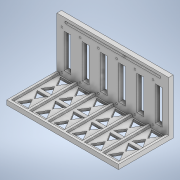
# Autodesk Inventor part: controllbox_1
Saved by Autodesk Inventor 2020 (Build 240168000, 168)
## iProperties
Created: 2020-05-26
Part Number: controllbox_1
Material: Generic
Document SubType Name: Modeling
Designer: Gebruiker
Density: 1 g/cm^3
Appearance: Default
Author: Gebruiker
Autodesk Inventor part; units mm, degrees
ref_plane "YZ Plane" through (0, 0, 0) normal (1, 0, 0) x (0, 1, 0)
ref_plane "XZ Plane" through (0, 0, 0) normal (0, 1, 0) x (-1, 0, 0)
ref_plane "XY Plane" through (0, 0, 0) normal (0, 0, 1) x (1, 0, 0)
sketch "Sketch1" plane through (0, 0, 0) normal (0, 0, 1) x (1, 0, 0)
  line L0 (-122.5, 60) -> (122.5, 60)
  line L1 (122.5, 60) -> (122.5, -60)
  line L2 (122.5, -60) -> (-122.5, -60)
  line L3 (-122.5, -60) -> (-122.5, 60)
  line L4 (-122.5, 60) -> (122.5, -60) construction
  line L5 (122.5, 60) -> (-122.5, -60) construction
  line L6 (-111.5, -60) -> (-111.5, 60) construction
  line L7 (-122.5, -47) -> (122.5, -47) construction
  circle A0 centre (-111.5, -47) radius 2
  circle A1 centre (-111.5, 39) radius 2
  line L8 (-111.5, 39) -> (122.5, 39) construction
  circle A2 centre (-71.5, -47) radius 2
  circle A3 centre (-31.5, -47) radius 2
  circle A4 centre (8.5, -47) radius 2
  circle A5 centre (48.5, -47) radius 2
  circle A6 centre (88.5, -47) radius 2
  line L9 (0, 60) -> (0, -60) construction
  circle A7 centre (-71.5, 39) radius 2
  circle A8 centre (-31.5, 39) radius 2
  circle A9 centre (8.5, 39) radius 2
  circle A10 centre (48.5, 39) radius 2
  circle A11 centre (88.5, 39) radius 2
  line L10 (-31.5, 39) -> (-31.5, -47) construction
  line L11 (-99.5, 60) -> (-99.5, -60) construction
  line L12 (-122.5, -4) -> (122.5, -4) construction
  line L13 (-107, 33.5) -> (-92, 33.5)
  line L14 (-92, 33.5) -> (-92, -41.5)
  line L15 (-92, -41.5) -> (-107, -41.5)
  line L16 (-107, -41.5) -> (-107, 33.5)
  line L17 (-107, 33.5) -> (-92, -41.5) construction
  line L18 (-92, 33.5) -> (-107, -41.5) construction
  line L19 (-67, 33.5) -> (-52, 33.5)
  line L20 (-52, 33.5) -> (-52, -41.5)
  line L21 (-67, -41.5) -> (-67, 33.5)
  line L22 (-52, -41.5) -> (-67, -41.5)
  line L23 (-27, 33.5) -> (-12, 33.5)
  line L24 (-12, 33.5) -> (-12, -41.5)
  line L25 (-27, -41.5) -> (-27, 33.5)
  line L26 (-12, -41.5) -> (-27, -41.5)
  line L27 (13, 33.5) -> (28, 33.5)
  line L28 (28, 33.5) -> (28, -41.5)
  line L29 (13, -41.5) -> (13, 33.5)
  line L30 (28, -41.5) -> (13, -41.5)
  line L31 (53, 33.5) -> (68, 33.5)
  line L32 (68, 33.5) -> (68, -41.5)
  line L33 (53, -41.5) -> (53, 33.5)
  line L34 (68, -41.5) -> (53, -41.5)
  line L35 (93, 33.5) -> (108, 33.5)
  line L36 (108, 33.5) -> (108, -41.5)
  line L37 (93, -41.5) -> (93, 33.5)
  line L38 (108, -41.5) -> (93, -41.5)
  line L39 (-105, 53.9067) -> (105, 53.9067)
  line L40 (105, 53.9067) -> (105, 48.9067)
  line L41 (105, 48.9067) -> (-105, 48.9067)
  line L42 (-105, 48.9067) -> (-105, 53.9067)
  line L43 (-105, 53.9067) -> (105, 48.9067) construction
  line L44 (105, 53.9067) -> (-105, 48.9067) construction
  point P0 (0, 0)
  point P1 (-99.5, -4)
  point P2 (0, 51.4067)
  dimension "d0" = 245
  dimension "d1" = 120
  dimension "d20" = 11
  dimension "d21" = 13
  dimension "d22" = 4
  dimension "d23" = 4
  dimension "d24" = 86
  dimension "d27" = 40
  dimension "d32" = 34
  dimension "d35" = 40
  dimension "d43" = 12
  dimension "d44" = 43
  dimension "d45" = 15
  dimension "d46" = 75
  dimension "d49" = 40
  dimension "d56" = 210
  dimension "d57" = 5
  constraints: 90 end point, 15 point on line, 12 centre point, 8 midpoint, 8 perpendicular, 6 horizontal, 6 parallel, 60 other
  measures "d0" distance of L1.end L2.end
  measures "d1" distance of L0.end L1.end
  measures "d20" distance between parallel lines of L6 L3
  measures "d21" distance between parallel lines of L7 L2
  measures "d22" diameter of A0
  measures "d23" diameter of A1
  measures "d24" distance of A0.centre L8.start
  measures "d27" distance of A0.centre A2.centre
  measures "d32" distance from line of L1 A6.centre
  measures "d35" distance of L8.start A7.centre
  measures "d43" distance from line of L11 L8.start
  measures "d44" distance from line of L12 L8.start
  measures "d45" distance of L14.end L15.end
  measures "d46" distance of L13.end L14.end
  measures "d49" distance of L13.start L19.start
  measures "d56" distance of L40.end L41.end
  measures "d57" distance of L39.end L40.end
extrude "Extrusion1" add sketch "Sketch1" against normal blind 10 contours L0 L1 L2 L3 | A0 | A1 | A2 | A3 | A4 | A5 | A6 | A7 | A8 | A9 | A10 | A11 | L13 L14 L15 L16 | L19 L20 L22 L21 | L23 L24 L26 L25 | L27 L28 L30 L29 | L31 L32 L34 L33 | L35 L36 L38 L37 | L39 L40 L41 L42
sketch "Sketch2" plane through (122.5, -60, 0) normal (1, 0, 0) x (0, 0, -1)
  line L0 (0, 0) -> (0, 120) projected
  line L1 (0, 0) -> (-110, 0)
  line L2 (-110, 0) -> (-110, 10)
  line L3 (-110, 10) -> (0, 10)
  line L4 (0, 10) -> (0, 0)
  point P0 (0, 60)
  dimension "d4" = 110
  dimension "d5" = 10
  constraints: 8 end point, 2 parallel, 1 horizontal, 1 perpendicular
  measures "d4" distance of L2.end L3.end
  measures "d5" distance of L1.end L2.end
extrude "Extrusion2" add sketch "Sketch2" against normal blind 245
sketch "Sketch3" plane through (122.5, -50, 110) normal (0, 1, 0) x (1, 0, 0)
  line L0 (0, 110) -> (-245, 110) projected
  line L1 (-240, 110) -> (-205, 110)
  line L2 (-205, 110) -> (-205, 5)
  line L3 (-205, 5) -> (-240, 5)
  line L4 (-240, 5) -> (-240, 110)
  line L5 (-245, 0) -> (-245, 110) projected
  line L6 (-245, 120) -> (-245, 0) projected
  line L7 (-245, 60) -> (0, 60) construction
  line L8 (0, 0) -> (0, 120) projected
  line L9 (-200, 110) -> (-165, 110)
  line L10 (-165, 110) -> (-165, 5)
  line L11 (-165, 5) -> (-200, 5)
  line L12 (-200, 5) -> (-200, 110)
  line L13 (-160, 110) -> (-125, 110)
  line L14 (-125, 110) -> (-125, 5)
  line L15 (-125, 5) -> (-160, 5)
  line L16 (-160, 5) -> (-160, 110)
  line L17 (-122.5, 110) -> (-122.5, 0) construction
  line L18 (0, 0) -> (-245, 0) construction
  line L19 (-40, 110) -> (-40, 5)
  line L20 (-40, 5) -> (-5, 5)
  line L21 (-5, 5) -> (-5, 110)
  line L22 (-80, 110) -> (-80, 5)
  line L23 (-80, 5) -> (-45, 5)
  line L24 (-45, 5) -> (-45, 110)
  line L25 (-120, 110) -> (-120, 5)
  line L26 (-120, 5) -> (-85, 5)
  line L27 (-85, 5) -> (-85, 110)
  line L28 (-234.4661, 12.7611) -> (-210.5339, 12.7611)
  line L29 (-210.5339, 12.7611) -> (-222.5, 33.6484)
  line L30 (-222.5, 33.6484) -> (-234.4661, 12.7611)
  line L31 (-222.5, 37.4721) -> (-234.4661, 56.2033)
  line L32 (-234.4661, 56.2033) -> (-210.5339, 56.2033)
  line L33 (-210.5339, 56.2033) -> (-222.5, 37.4721)
  line L34 (-210.5339, 107.2389) -> (-222.5, 86.3516)
  line L35 (-222.5, 86.3516) -> (-234.4661, 107.2389)
  line L36 (-222.5, 82.5279) -> (-234.4661, 63.7967)
  line L37 (-234.4661, 63.7967) -> (-210.5339, 63.7967)
  line L38 (-210.5339, 63.7967) -> (-222.5, 82.5279)
  line L39 (-234.4661, 107.2389) -> (-210.5339, 107.2389)
  line L40 (-205, 110) -> (-200, 110) construction
  line L41 (-200, 110) -> (-200, 5) construction
  line L42 (-200, 5) -> (-205, 5) construction
  line L43 (-205, 5) -> (-205, 110) construction
  line L44 (-202.5, 110) -> (-202.5, 5) construction
  line L45 (-170.5339, 12.7611) -> (-194.4661, 12.7611)
  line L46 (-194.4661, 12.7611) -> (-182.5, 33.6484)
  line L47 (-182.5, 33.6484) -> (-170.5339, 12.7611)
  line L48 (-182.5, 37.4721) -> (-170.5339, 56.2033)
  line L49 (-170.5339, 56.2033) -> (-194.4661, 56.2033)
  line L50 (-194.4661, 56.2033) -> (-182.5, 37.4721)
  line L51 (-194.4661, 63.7967) -> (-182.5, 82.5279)
  line L52 (-170.5339, 63.7967) -> (-194.4661, 63.7967)
  line L53 (-182.5, 82.5279) -> (-170.5339, 63.7967)
  line L54 (-182.5, 86.3516) -> (-170.5339, 107.2389)
  line L55 (-194.4661, 107.2389) -> (-182.5, 86.3516)
  line L56 (-170.5339, 107.2389) -> (-194.4661, 107.2389)
  line L57 (-165, 110) -> (-160, 110) construction
  line L58 (-160, 110) -> (-160, 5) construction
  line L59 (-160, 5) -> (-165, 5) construction
  line L60 (-165, 5) -> (-165, 110) construction
  line L61 (-162.5, 110) -> (-162.5, 5) construction
  line L62 (-130.5339, 12.7611) -> (-142.5, 33.6484)
  line L63 (-142.5, 33.6484) -> (-154.4661, 12.7611)
  line L64 (-154.4661, 12.7611) -> (-130.5339, 12.7611)
  line L65 (-142.5, 37.4721) -> (-154.4661, 56.2033)
  line L66 (-130.5339, 56.2033) -> (-142.5, 37.4721)
  line L67 (-154.4661, 56.2033) -> (-130.5339, 56.2033)
  line L68 (-154.4661, 63.7967) -> (-130.5339, 63.7967)
  line L69 (-130.5339, 63.7967) -> (-142.5, 82.5279)
  line L70 (-142.5, 82.5279) -> (-154.4661, 63.7967)
  line L71 (-142.5, 86.3516) -> (-154.4661, 107.2389)
  line L72 (-130.5339, 107.2389) -> (-142.5, 86.3516)
  line L73 (-154.4661, 107.2389) -> (-130.5339, 107.2389)
  line L74 (-10.5339, 12.7611) -> (-34.4661, 12.7611)
  line L75 (-22.5, 33.6484) -> (-10.5339, 12.7611)
  line L76 (-22.5, 37.4721) -> (-10.5339, 56.2033)
  line L77 (-10.5339, 56.2033) -> (-34.4661, 56.2033)
  line L78 (-34.4661, 56.2033) -> (-22.5, 37.4721)
  line L79 (-34.4661, 63.7967) -> (-22.5, 82.5279)
  line L80 (-10.5339, 63.7967) -> (-34.4661, 63.7967)
  line L81 (-22.5, 82.5279) -> (-10.5339, 63.7967)
  line L82 (-22.5, 86.3516) -> (-10.5339, 107.2389)
  line L83 (-34.4661, 107.2389) -> (-22.5, 86.3516)
  line L84 (-10.5339, 107.2389) -> (-34.4661, 107.2389)
  line L85 (-50.5339, 12.7611) -> (-62.5, 33.6484)
  line L86 (-74.4661, 12.7611) -> (-50.5339, 12.7611)
  line L87 (-62.5, 37.4721) -> (-74.4661, 56.2033)
  line L88 (-50.5339, 56.2033) -> (-62.5, 37.4721)
  line L89 (-74.4661, 56.2033) -> (-50.5339, 56.2033)
  line L90 (-74.4661, 63.7967) -> (-50.5339, 63.7967)
  line L91 (-50.5339, 63.7967) -> (-62.5, 82.5279)
  line L92 (-62.5, 82.5279) -> (-74.4661, 63.7967)
  line L93 (-62.5, 86.3516) -> (-74.4661, 107.2389)
  line L94 (-50.5339, 107.2389) -> (-62.5, 86.3516)
  line L95 (-74.4661, 107.2389) -> (-50.5339, 107.2389)
  line L96 (-102.5, 33.6484) -> (-90.5339, 12.7611)
  line L97 (-90.5339, 12.7611) -> (-114.4661, 12.7611)
  line L98 (-114.4661, 12.7611) -> (-102.5, 33.6484)
  line L99 (-114.4661, 56.2033) -> (-102.5, 37.4721)
  line L100 (-102.5, 37.4721) -> (-90.5339, 56.2033)
  line L101 (-90.5339, 56.2033) -> (-114.4661, 56.2033)
  line L102 (-90.5339, 63.7967) -> (-114.4661, 63.7967)
  line L103 (-102.5, 82.5279) -> (-90.5339, 63.7967)
  line L104 (-114.4661, 63.7967) -> (-102.5, 82.5279)
  line L105 (-114.4661, 107.2389) -> (-102.5, 86.3516)
  line L106 (-102.5, 86.3516) -> (-90.5339, 107.2389)
  line L107 (-90.5339, 107.2389) -> (-114.4661, 107.2389)
  line L108 (-74.4661, 12.7611) -> (-62.5, 33.6484)
  line L109 (-34.4661, 12.7611) -> (-22.5, 33.6484)
  dimension "d8" = 35
  dimension "d9" = 105
  dimension "d10" = 5
  dimension "d11" = 35
  dimension "d12" = 35
  dimension "d13" = 105
  dimension "d14" = 5
  dimension "d15" = 5
  constraints: 210 end point, 78 symmetric about line, 10 parallel, 8 horizontal, 7 midpoint, 5 perpendicular, 3 equal length, 3 point on line
  measures "d8" distance of L2.end L3.end
  measures "d9" distance of L1.end L2.end
  measures "d10" distance between parallel lines of L4 L5
  measures "d11" distance of L10.end L11.end
  measures "d12" distance of L14.end L15.end
  measures "d13" distance of L13.end L14.end
  measures "d14" distance between parallel lines of L12 L2
  measures "d15" distance between parallel lines of L16 L10
extrude "Extrusion3" cut sketch "Sketch3" against normal blind 5 contours L21 L20 L19 L0 | L2 L3 L4 L0 | L10 L11 L12 L0 | L14 L15 L16 L0 | L27 L26 L25 L0 | L24 L23 L22 L0 | L30 L29 L28 | L31 L32 L33 | L34 L35 L39 | L38 L37 L36 | L45 L46 L47 | L50 L49 L48 | L51 L53 L52 | L55 L56 L54 | L64 L63 L62 | L65 L67 L66 | L70 L69 L68 | L71 L73 L72 | L74 L109 L75 | L78 L77 L76 | L79 L81 L80 | L83 L84 L82 | L86 L108 L85 | L87 L89 L88 | L92 L91 L90 | L93 L95 L94 | L96 L97 L98 | L101 L100 L99 | L102 L104 L103 | L107 L106 L105
extrude "Extrusion4" cut sketch "Sketch3" against normal blind 10 contours L30 L29 L28 | L31 L32 L33 | L34 L35 L39 | L38 L37 L36 | L45 L46 L47 | L50 L49 L48 | L51 L53 L52 | L55 L56 L54 | L64 L63 L62 | L65 L67 L66 | L70 L69 L68 | L71 L73 L72 | L74 L109 L75 | L78 L77 L76 | L79 L81 L80 | L83 L84 L82 | L86 L108 L85 | L87 L89 L88 | L92 L91 L90 | L93 L95 L94 | L96 L97 L98 | L101 L100 L99 | L102 L104 L103 | L107 L106 L105
extrude "Extrusion5" cut sketch "Sketch1" against normal blind 10 contours A0 | A1 | A2 | A3 | A4 | A5 | A6 | A7 | A8 | A9 | A10 | A11
extrude "Extrusion6" cut sketch "Sketch1" against normal blind 10 contours L13 L14 L15 L16 | L19 L20 L22 L21 | L23 L24 L26 L25 | L27 L28 L30 L29 | L31 L32 L34 L33 | L35 L36 L38 L37
extrude "Extrusion7" cut sketch "Sketch1" against normal blind 10 contours L39 L40 L41 L42
fillet "Fillet1" radius 2 4 edges at (-105, 48.9067, -5) (-105, 53.9067, -5) (105, 48.9067, -5) (105, 53.9067, -5)
body "Solid1"
